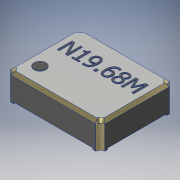
# Autodesk Inventor part: Crystal_TXO-3225
Saved by Autodesk Inventor 2018 (Build 220112000, 112)
## iProperties
Created: 2016-08-15
Part Number: Crystal_TXO-3225
Material: Aluminum 6061
Document SubType Name: Modeling
Designer: Bradley
Density: 2.7 g/cm^3
Appearance: Aluminum - Flat
Author: Bradley
Autodesk Inventor part; units mm, degrees
ref_plane "YZ Plane" through (0, 0, 0) normal (1, 0, 0) x (0, 1, 0)
ref_plane "XZ Plane" through (0, 0, 0) normal (0, 1, 0) x (-1, 0, 0)
ref_plane "XY Plane" through (0, 0, 0) normal (0, 0, 1) x (1, 0, 0)
sketch "Sketch1" plane through (0, 0, 0) normal (0, 1, 0) x (-1, 0, 0)
  line L0 (-1.6, 1.25) -> (1.6, 1.25)
  line L1 (1.6, 1.25) -> (1.6, -1.25)
  line L2 (1.6, -1.25) -> (-1.6, -1.25)
  line L3 (-1.6, -1.25) -> (-1.6, 1.25)
  line L4 (-1.6, 1.25) -> (1.6, -1.25) construction
  line L5 (1.6, 1.25) -> (-1.6, -1.25) construction
  arc A0 (1.6, -1.1) -> (1.45, -1.25) centre (1.6, -1.25) ccw
  arc A1 (-1.45, -1.25) -> (-1.6, -1.1) centre (-1.6, -1.25) ccw
  arc A2 (-1.6, 1.1) -> (-1.45, 1.25) centre (-1.6, 1.25) ccw
  arc A3 (1.45, 1.25) -> (1.6, 1.1) centre (1.6, 1.25) ccw
  point P0 (0, 0)
  dimension "d0" = 3.2
  dimension "d1" = 2.5
  dimension "d4" = 0.15
  constraints: 12 end point, 8 point on circle, 8 point on line, 4 centre point, 4 coincident, 3 equal radius, 2 midpoint, 2 parallel, 1 horizontal, 1 perpendicular
  measures "d0" distance of L1.end L2.end
  measures "d1" distance of L0.end L1.end
  measures "d4" radius of A0
extrude "Extrusion1" add sketch "Sketch1" along normal mid plane 0.85 contours L0 A3 L1 A0 L2 A1 L3 A2
chamfer "Chamfer1" distance 0.1 angle 45 8 edges at (0, 0.425, 1.25) (-1.4939, 0.425, 1.1439) (-1.6, 0.425, 0) (-1.4939, 0.425, -1.1439) (0, 0.425, -1.25) (1.4939, 0.425, -1.1439) (1.6, 0.425, 0) (1.4939, 0.425, 1.1439)
sketch "Sketch3" plane through (0, 0.425, 0) normal (0, 1, 0) x (1, 0, 0)
  line L0 (-1.3709, 1.15) -> (1.3709, 1.15) projected
  arc A0 (-1.5, 1.0209) -> (-1.3709, 1.15) centre (-1.6, 1.25) ccw projected
  line L1 (-1.5, -1.0209) -> (-1.5, 1.0209) projected
  arc A1 (-1.3709, -1.15) -> (-1.5, -1.0209) centre (-1.6, -1.25) ccw projected
  line L2 (1.3709, -1.15) -> (-1.3709, -1.15) projected
  arc A2 (1.5, -1.0209) -> (1.3709, -1.15) centre (1.6, -1.25) ccw projected
  line L3 (1.5, 1.0209) -> (1.5, -1.0209) projected
  arc A3 (1.3709, 1.15) -> (1.5, 1.0209) centre (1.6, 1.25) ccw projected
  line L4 (1.5, 1.0209) -> (1.5, -1.0209) construction
  line L5 (1.5, 0.1868) -> (-1.5, 0.1868) construction
  circle A4 centre (-1.1, -0.6) radius 0.2
  line L6 (-0.9406, 0.1868) -> (-1.0152, 0.1868)
  line L7 (-1.0152, 0.1868) -> (-1.2364, 0.6179)
  line L8 (-1.2364, 0.6179) -> (-1.2364, 0.1868)
  line L9 (-1.2364, 0.1868) -> (-1.2984, 0.1868)
  line L10 (-1.2984, 0.1868) -> (-1.2984, 0.6868)
  line L11 (-1.2984, 0.6868) -> (-1.204, 0.6868)
  line L12 (-1.204, 0.6868) -> (-1.0026, 0.2909)
  line L13 (-1.0026, 0.2909) -> (-1.0026, 0.6868)
  line L14 (-1.0026, 0.6868) -> (-0.9406, 0.6868)
  line L15 (-0.9406, 0.6868) -> (-0.9406, 0.1868)
  line L16 (-0.5703, 0.1868) -> (-0.8142, 0.1868)
  line L17 (-0.8142, 0.1868) -> (-0.8142, 0.2378)
  line L18 (-0.8142, 0.2378) -> (-0.7235, 0.2378)
  line L19 (-0.7235, 0.2378) -> (-0.7235, 0.5729)
  line L20 (-0.7235, 0.5729) -> (-0.8142, 0.5729)
  line L21 (-0.8142, 0.5729) -> (-0.8142, 0.6187)
  spline S0 degree 2 poles (-0.8142, 0.6187) (-0.7628, 0.6187) (-0.7141, 0.6479) (-0.7109, 0.6884) knots 0 0 0 1 2 2 2
  line L22 (-0.7109, 0.6884) -> (-0.659, 0.6884)
  line L23 (-0.659, 0.6884) -> (-0.659, 0.2378)
  line L24 (-0.659, 0.2378) -> (-0.5703, 0.2378)
  line L25 (-0.5703, 0.2378) -> (-0.5703, 0.1868)
  spline S1 degree 2 poles (-0.4921, 0.5243) (-0.4921, 0.5628) (-0.467, 0.6268) (-0.4451, 0.6499) knots 0 0 0 1 2 2 2
  spline S2 degree 2 poles (-0.4451, 0.6499) (-0.4244, 0.6722) (-0.3641, 0.6969) (-0.3333, 0.6969) knots 0 0 0 1 2 2 2
  spline S3 degree 2 poles (-0.3333, 0.6969) (-0.2988, 0.6969) (-0.2429, 0.6738) (-0.2222, 0.6519) knots 0 0 0 1 2 2 2
  spline S4 degree 2 poles (-0.2222, 0.6519) (-0.1963, 0.6244) (-0.1679, 0.5352) (-0.1679, 0.4667) knots 0 0 0 1 2 2 2
  spline S5 degree 2 poles (-0.1679, 0.4667) (-0.1679, 0.4047) (-0.1959, 0.2937) (-0.2231, 0.2569) knots 0 0 0 1 2 2 2
  spline S6 degree 2 poles (-0.2231, 0.2569) (-0.2518, 0.218) (-0.3329, 0.177) (-0.392, 0.177) knots 0 0 0 1 2 2 2
  spline S7 degree 2 poles (-0.392, 0.177) (-0.4054, 0.177) (-0.4358, 0.1799) (-0.4487, 0.1839) knots 0 0 0 1 2 2 2
  line L26 (-0.4487, 0.1839) -> (-0.4487, 0.2483)
  line L27 (-0.4487, 0.2483) -> (-0.4455, 0.2483)
  spline S8 degree 2 poles (-0.4455, 0.2483) (-0.437, 0.2435) (-0.4013, 0.235) (-0.3831, 0.235) knots 0 0 0 1 2 2 2
  spline S9 degree 2 poles (-0.3831, 0.235) (-0.3175, 0.235) (-0.2425, 0.3217) (-0.2372, 0.4019) knots 0 0 0 1 2 2 2
  spline S10 degree 2 poles (-0.2372, 0.4019) (-0.264, 0.3837) (-0.3126, 0.3671) (-0.3414, 0.3671) knots 0 0 0 1 2 2 2
  spline S11 degree 2 poles (-0.3414, 0.3671) (-0.3689, 0.3671) (-0.4147, 0.3792) (-0.4378, 0.3966) knots 0 0 0 1 2 2 2
  spline S12 degree 2 poles (-0.4378, 0.3966) (-0.4645, 0.4173) (-0.4921, 0.4801) (-0.4921, 0.5243) knots 0 0 0 1 2 2 2
  spline S13 degree 2 poles (-0.2356, 0.4817) (-0.2356, 0.5324) (-0.2543, 0.5964) (-0.2709, 0.6138) knots 0 0 0 1 2 2 2
  spline S14 degree 2 poles (-0.2709, 0.6138) (-0.2855, 0.63) (-0.3158, 0.6422) (-0.3337, 0.6422) knots 0 0 0 1 2 2 2
  spline S15 degree 2 poles (-0.3337, 0.6422) (-0.375, 0.6422) (-0.424, 0.583) (-0.424, 0.5271) knots 0 0 0 1 2 2 2
  spline S16 degree 2 poles (-0.424, 0.5271) (-0.424, 0.4955) (-0.4078, 0.4546) (-0.39, 0.44) knots 0 0 0 1 2 2 2
  spline S17 degree 2 poles (-0.39, 0.44) (-0.377, 0.4295) (-0.345, 0.4226) (-0.3264, 0.4226) knots 0 0 0 1 2 2 2
  spline S18 degree 2 poles (-0.3264, 0.4226) (-0.3049, 0.4226) (-0.2555, 0.4376) (-0.2368, 0.4501) knots 0 0 0 1 2 2 2
  spline S19 degree 2 poles (-0.2368, 0.4501) (-0.2364, 0.455) (-0.2356, 0.4716) (-0.2356, 0.4817) knots 0 0 0 1 2 2 2
  line L28 (0.0043, 0.1868) -> (-0.076, 0.1868)
  line L29 (-0.076, 0.1868) -> (-0.076, 0.2824)
  line L30 (-0.076, 0.2824) -> (0.0043, 0.2824)
  line L31 (0.0043, 0.2824) -> (0.0043, 0.1868)
  spline S20 degree 2 poles (0.4212, 0.3488) (0.4212, 0.3103) (0.3957, 0.2451) (0.3742, 0.2232) knots 0 0 0 1 2 2 2
  spline S21 degree 2 poles (0.3742, 0.2232) (0.3519, 0.2001) (0.296, 0.1762) (0.2624, 0.1762) knots 0 0 0 1 2 2 2
  spline S22 degree 2 poles (0.2624, 0.1762) (0.2287, 0.1762) (0.1732, 0.1989) (0.1521, 0.2216) knots 0 0 0 1 2 2 2
  spline S23 degree 2 poles (0.1521, 0.2216) (0.1262, 0.2488) (0.097, 0.3399) (0.097, 0.4064) knots 0 0 0 1 2 2 2
  spline S24 degree 2 poles (0.097, 0.4064) (0.097, 0.4716) (0.1238, 0.5765) (0.1517, 0.6154) knots 0 0 0 1 2 2 2
  spline S25 degree 2 poles (0.1517, 0.6154) (0.1789, 0.6535) (0.2648, 0.6961) (0.3211, 0.6961) knots 0 0 0 1 2 2 2
  spline S26 degree 2 poles (0.3211, 0.6961) (0.3377, 0.6961) (0.3669, 0.6928) (0.3778, 0.6892) knots 0 0 0 1 2 2 2
  line L32 (0.3778, 0.6892) -> (0.3778, 0.6248)
  line L33 (0.3778, 0.6248) -> (0.375, 0.6248)
  spline S27 degree 2 poles (0.375, 0.6248) (0.3657, 0.6296) (0.3316, 0.6381) (0.3122, 0.6381) knots 0 0 0 1 2 2 2
  spline S28 degree 2 poles (0.3122, 0.6381) (0.2498, 0.6381) (0.1732, 0.5539) (0.1659, 0.4712) knots 0 0 0 1 2 2 2
  spline S29 degree 2 poles (0.1659, 0.4712) (0.1898, 0.4878) (0.2401, 0.506) (0.2701, 0.506) knots 0 0 0 1 2 2 2
  spline S30 degree 2 poles (0.2701, 0.506) (0.2992, 0.506) (0.343, 0.4943) (0.3669, 0.4765) knots 0 0 0 1 2 2 2
  spline S31 degree 2 poles (0.3669, 0.4765) (0.3944, 0.4558) (0.4212, 0.3918) (0.4212, 0.3488) knots 0 0 0 1 2 2 2
  spline S32 degree 2 poles (0.3531, 0.346) (0.3531, 0.3768) (0.3369, 0.4185) (0.3191, 0.4331) knots 0 0 0 1 2 2 2
  spline S33 degree 2 poles (0.3191, 0.4331) (0.3057, 0.4436) (0.2725, 0.4505) (0.2551, 0.4505) knots 0 0 0 1 2 2 2
  spline S34 degree 2 poles (0.2551, 0.4505) (0.2316, 0.4505) (0.1874, 0.4364) (0.1659, 0.423) knots 0 0 0 1 2 2 2
  spline S35 degree 2 poles (0.1659, 0.423) (0.1655, 0.4157) (0.1647, 0.4019) (0.1647, 0.3914) knots 0 0 0 1 2 2 2
  spline S36 degree 2 poles (0.1647, 0.3914) (0.1647, 0.3395) (0.185, 0.2759) (0.2004, 0.2593) knots 0 0 0 1 2 2 2
  spline S37 degree 2 poles (0.2004, 0.2593) (0.2145, 0.2435) (0.2453, 0.2309) (0.2628, 0.2309) knots 0 0 0 1 2 2 2
  spline S38 degree 2 poles (0.2628, 0.2309) (0.3033, 0.2309) (0.3531, 0.2885) (0.3531, 0.346) knots 0 0 0 1 2 2 2
  spline S39 degree 2 poles (0.6315, 0.1754) (0.5942, 0.1754) (0.533, 0.1977) (0.5115, 0.2184) knots 0 0 0 1 2 2 2
  spline S40 degree 2 poles (0.5115, 0.2184) (0.4905, 0.2386) (0.4686, 0.2937) (0.4686, 0.3249) knots 0 0 0 1 2 2 2
  spline S41 degree 2 poles (0.4686, 0.3249) (0.4686, 0.3654) (0.512, 0.4335) (0.5533, 0.4538) knots 0 0 0 1 2 2 2
  line L34 (0.5533, 0.4538) -> (0.5533, 0.4558)
  spline S42 degree 2 poles (0.5533, 0.4558) (0.5164, 0.4773) (0.4808, 0.5283) (0.4808, 0.5664) knots 0 0 0 1 2 2 2
  spline S43 degree 2 poles (0.4808, 0.5664) (0.4808, 0.6227) (0.5658, 0.6981) (0.6315, 0.6981) knots 0 0 0 1 2 2 2
  spline S44 degree 2 poles (0.6315, 0.6981) (0.6996, 0.6981) (0.7818, 0.6268) (0.7818, 0.5709) knots 0 0 0 1 2 2 2
  spline S45 degree 2 poles (0.7818, 0.5709) (0.7818, 0.5372) (0.7425, 0.4716) (0.7056, 0.453) knots 0 0 0 1 2 2 2
  line L35 (0.7056, 0.453) -> (0.7056, 0.4509)
  spline S46 degree 2 poles (0.7056, 0.4509) (0.7494, 0.4307) (0.7944, 0.3723) (0.7944, 0.3261) knots 0 0 0 1 2 2 2
  spline S47 degree 2 poles (0.7944, 0.3261) (0.7944, 0.2621) (0.7012, 0.1754) (0.6315, 0.1754) knots 0 0 0 1 2 2 2
  spline S48 degree 2 poles (0.7255, 0.3197) (0.7255, 0.3505) (0.7012, 0.3869) (0.6667, 0.4056) knots 0 0 0 1 2 2 2
  spline S49 degree 2 poles (0.6667, 0.4056) (0.6554, 0.412) (0.6173, 0.427) (0.5934, 0.4368) knots 0 0 0 1 2 2 2
  spline S50 degree 2 poles (0.5934, 0.4368) (0.5658, 0.4185) (0.5363, 0.3642) (0.5363, 0.3298) knots 0 0 0 1 2 2 2
  spline S51 degree 2 poles (0.5363, 0.3298) (0.5363, 0.2844) (0.591, 0.2252) (0.6323, 0.2252) knots 0 0 0 1 2 2 2
  spline S52 degree 2 poles (0.6323, 0.2252) (0.6744, 0.2252) (0.7255, 0.2759) (0.7255, 0.3197) knots 0 0 0 1 2 2 2
  spline S53 degree 2 poles (0.7162, 0.5701) (0.7162, 0.6037) (0.6712, 0.6487) (0.6311, 0.6487) knots 0 0 0 1 2 2 2
  spline S54 degree 2 poles (0.6311, 0.6487) (0.5946, 0.6487) (0.548, 0.6086) (0.548, 0.5741) knots 0 0 0 1 2 2 2
  spline S55 degree 2 poles (0.548, 0.5741) (0.548, 0.5494) (0.5719, 0.515) (0.5958, 0.5012) knots 0 0 0 1 2 2 2
  spline S56 degree 2 poles (0.5958, 0.5012) (0.606, 0.4955) (0.6489, 0.4757) (0.6663, 0.47) knots 0 0 0 1 2 2 2
  spline S57 degree 2 poles (0.6663, 0.47) (0.6955, 0.4923) (0.7162, 0.5397) (0.7162, 0.5701) knots 0 0 0 1 2 2 2
  line L36 (1.2984, 0.1868) -> (1.232, 0.1868)
  line L37 (1.232, 0.1868) -> (1.232, 0.6175)
  line L38 (1.232, 0.6175) -> (1.1015, 0.3245)
  line L39 (1.1015, 0.3245) -> (1.061, 0.3245)
  line L40 (1.061, 0.3245) -> (0.9317, 0.6175)
  line L41 (0.9317, 0.6175) -> (0.9317, 0.1868)
  line L42 (0.9317, 0.1868) -> (0.8697, 0.1868)
  line L43 (0.8697, 0.1868) -> (0.8697, 0.6868)
  line L44 (0.8697, 0.6868) -> (0.9605, 0.6868)
  line L45 (0.9605, 0.6868) -> (1.0853, 0.4084)
  line L46 (1.0853, 0.4084) -> (1.206, 0.6868)
  line L47 (1.206, 0.6868) -> (1.2984, 0.6868)
  line L48 (1.2984, 0.6868) -> (1.2984, 0.1868)
  point P0 (0, 0)
  dimension "d27" = 0.4
  dimension "d28" = 0.6
  dimension "d29" = 1.1
  constraints: 2 end point, 2 point on line, 1 centre point, 1 horizontal, 1 perpendicular
  measures "d27" diameter of A4
  measures "d28" vertical distance of point (0, 0) A4.centre
  measures "d29" horizontal distance of point (0, 0) A4.centre
extrude "Extrusion3" add sketch "Sketch3" along normal blind 0.01 contours A4 | L6 L7 L8 L9 L10 L11 L12 L13 L14 L15 | L16 L17 L18 L19 L20 L21 S0 L22 L23 L24 L25 | S1 S2 S3 S4 S5 S6 S7 L26 L27 S8 S9 S10 S11 S12 | L28 L29 L30 L31 | S20 S21 S22 S23 S24 S25 S26 L32 L33 S27 S28 S29 S30 S31 | S39 S40 S41 S42 S43 S44 S45 L35 S46 S47 | L36 L37 L38 L39 L40 L41 L42 L43 L44 L45 L46 L47 L48
sketch "Sketch4" plane through (0, -0.425, 0) normal (0, -1, 0) x (1, 0, 0)
  line L0 (-1.6, 1.1) -> (-1.6, -1.1) projected
  arc A0 (-1.45, -1.25) -> (-1.6, -1.1) centre (-1.6, -1.25) ccw projected
  line L1 (-1.45, -1.25) -> (1.45, -1.25) projected
  arc A1 (1.6, -1.1) -> (1.45, -1.25) centre (1.6, -1.25) ccw projected
  line L2 (1.6, -1.1) -> (1.6, 1.1) projected
  arc A2 (1.45, 1.25) -> (1.6, 1.1) centre (1.6, 1.25) ccw projected
  line L3 (1.45, 1.25) -> (-1.45, 1.25) projected
  arc A3 (-1.6, 1.1) -> (-1.45, 1.25) centre (-1.6, 1.25) ccw projected
  line L4 (1.35, 1.25) -> (1.35, 1.19)
  line L5 (1.35, 1.19) -> (0.94, 1.19)
  line L6 (0.94, 1.19) -> (0.94, 0.35)
  line L7 (0.94, 0.35) -> (1.54, 0.35)
  line L8 (1.54, 0.35) -> (1.54, 1)
  line L9 (1.54, 1) -> (1.6, 1)
  line L10 (-1.6, -1.1) -> (-1.6, 1.1) projected
  line L11 (-1.6, 1) -> (-1.54, 1)
  line L12 (-1.54, 1) -> (-1.54, 0.35)
  line L13 (-1.54, 0.35) -> (-0.94, 0.35)
  line L14 (-0.94, 0.35) -> (-0.94, 1.19)
  line L15 (-0.94, 1.19) -> (-1.35, 1.19)
  line L16 (-1.35, 1.19) -> (-1.35, 1.25)
  line L17 (1.45, -1.25) -> (-1.45, -1.25) projected
  line L18 (-1.35, -1.25) -> (-1.35, -1.19)
  line L19 (-1.35, -1.19) -> (-0.94, -1.19)
  line L20 (-0.94, -1.19) -> (-0.94, -0.35)
  line L21 (-0.94, -0.35) -> (-1.54, -0.35)
  line L22 (-1.54, -0.35) -> (-1.54, -1)
  line L23 (-1.54, -1) -> (-1.6, -1)
  line L24 (1.6, -1) -> (1.54, -1)
  line L25 (1.54, -1) -> (1.54, -0.35)
  line L26 (1.54, -0.35) -> (0.94, -0.35)
  line L27 (0.94, -0.35) -> (0.94, -1.19)
  line L28 (0.94, -1.19) -> (1.35, -1.19)
  line L29 (1.35, -1.19) -> (1.35, -1.25)
  point P0 (0, 0)
  dimension "d20" = 0.84
  dimension "d21" = 0.6
  dimension "d22" = 1.88
  dimension "d23" = 0.25
  dimension "d24" = 0.25
  constraints: 48 end point, 20 point on line, 15 perpendicular, 7 equal length, 6 collinear, 1 horizontal, 1 parallel, 1 vertical
  measures "d20" distance of L5.end L6.end
  measures "d21" distance of L6.end L7.end
  measures "d22" distance between parallel lines of L14 L6
  measures "d23" distance between parallel lines of L4 L2
  measures "d24" distance between parallel lines of L9 L3
extrude "Extrusion5" add sketch "Sketch4" along normal blind 0.05 contours A3 L3 L16 L15 L14 L13 L12 L11 L0 | L23 L22 L21 L20 L19 L18 L1 A0 L0 | L3 A2 L2 L9 L8 L7 L6 L5 L4 | L29 L28 L27 L26 L25 L24 L2 A1 L1
equation "\"d24\" = d23"
body "Solid1"
